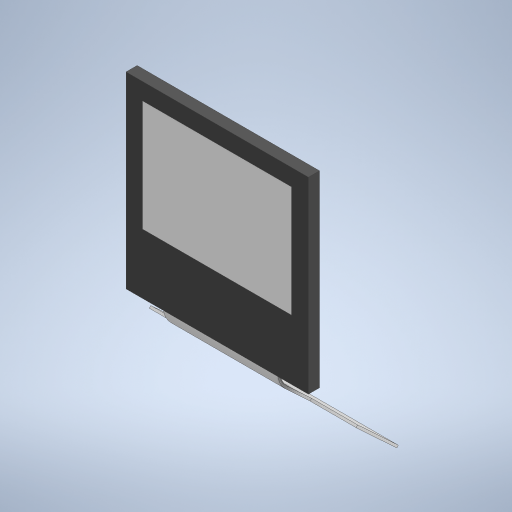
# Autodesk Inventor part: 0_42_oled
Saved by Autodesk Inventor 2023 (Build 270158000, 158)
## iProperties
Created: 2024-03-19
Part Number: 0_42_oled
Material: Generic
Document SubType Name: Modeling
Designer: noname
Density: 1 g/cm^3
Appearance: Default
Author: noname
Autodesk Inventor part; units mm, degrees
ref_plane "YZ Plane" through (0, 0, 0) normal (1, 0, 0) x (0, 1, 0)
ref_plane "XZ Plane" through (0, 0, 0) normal (0, 1, 0) x (-1, 0, 0)
ref_plane "XY Plane" through (0, 0, 0) normal (0, 0, 1) x (1, 0, 0)
sketch "Sketch2" plane through (0, 0, 0) normal (0, 0, 1) x (1, 0, 0)
  line L0 (-8.2, 0) -> (8.2, 0)
  line L1 (8.2, 0) -> (8.2, 16.9)
  line L2 (8.2, 16.9) -> (-8.2, 16.9)
  line L3 (-8.2, 16.9) -> (-8.2, 0)
  point P0 (0, 0)
  point P1 (0, 0)
  dimension "d0" = 16.4
  dimension "d1" = 16.9
  constraints: 8 end point, 2 parallel, 1 coincident, 1 horizontal, 1 midpoint, 1 perpendicular
  measures "d0" distance between parallel lines of L1 L3
  measures "d1" distance between parallel lines of L0 L2
extrude "Extrusion1" add sketch "Sketch2" along normal blind 1
ref_plane "Work Plane1" through (0, 0, 0.25) normal (0, 0, -1) x (-1, 0, 0)
sketch "Sketch5" plane through (0, 0, 0) normal (0, 0, -1) x (-1, 0, 0)
  line L0 (-6.7, 5.4) -> (6.7, 5.4)
  line L1 (6.7, 5.4) -> (6.7, 15.4)
  line L2 (6.7, 15.4) -> (-6.7, 15.4)
  line L3 (-6.7, 15.4) -> (-6.7, 5.4)
  line L4 (8.2, 16.9) -> (8.2, 0) projected
  line L5 (8.2, 0) -> (-8.2, 0) projected
  line L6 (-8.2, 16.9) -> (8.2, 16.9) projected
  point P0 (0, 0)
  point P1 (0, 5.4)
  point P2 (0, 0)
  dimension "d13" = 10
  dimension "d15" = 1.5
  dimension "d16" = 1.5
  constraints: 8 end point, 2 midpoint, 2 parallel, 1 horizontal, 1 perpendicular, 1 vertical alignment
  measures "d13" distance between parallel lines of L2 L0
  measures "d15" distance between parallel lines of L4 L1
  measures "d16" distance between parallel lines of L6 L2
ref_plane "Work Plane2" through (0, 0, 0) normal (1, 0, 0) x (0, 0, -1)
sketch "Sketch7" plane through (0, 0, 0) normal (1, 0, 0) x (0, 0, -1)
  arc A0 (-0.5, 0) -> (0.136, -1.4627) centre (1.5, 0) ccw
  line L0 (0, 0) -> (-1, 0) projected
  line L1 (0.136, -1.4627) -> (5.9868, -6.9187)
  line L2 (0, 16.9) -> (0, 0) projected
  line L3 (5.8504, -7.065) -> (-0.0004, -1.609)
  arc A1 (-0.7, 0) -> (-0.0004, -1.609) centre (1.5, 0) ccw
  line L4 (5.8504, -7.065) -> (5.9868, -6.9187)
  point P0 (5.9186, -6.9918)
  dimension "d19" = 2
  dimension "d22" = 43
  dimension "d23" = 0.5
  dimension "d24" = 0.2
  dimension "d33" = 8
  constraints: 6 end point, 4 point on circle, 2 centre point, 2 midpoint, 1 line through centre, 1 perpendicular, 1 point on line, 1 tangent, 1 other
  measures "d19" radius of A0
  measures "d22" angle of L0 L1
  measures "d23" distance from line of L2 A0.start
  measures "d24" distance between parallel lines of L1 L3
  measures "d33" distance of L1.start L1.end
extrude "Extrusion4" add sketch "Sketch7" along normal mid plane 10.3
sketch "Sketch8" plane through (0, 0, 0) normal (1, 0, 0) x (0, 0, -1)
  arc A0 (-0.5, 0) -> (0.136, -1.4627) centre (1.5, 0) ccw projected
  line L0 (-0.7, 0) -> (-0.5, 0) projected
  arc A1 (-0.7, 0) -> (-0.0004, -1.609) centre (1.5, 0) ccw construction
  line L1 (-0.0004, -1.609) -> (5.8504, -7.065) projected
  line L2 (5.8504, -7.065) -> (5.9868, -6.9187) projected
  line L3 (5.9868, -6.9187) -> (0.136, -1.4627) projected
  line L4 (2.1937, -3.655) -> (2.3301, -3.5087)
  point P0 (0, 0)
  dimension "d28" = 5
  constraints: 2 end point, 2 point on line, 1 perpendicular
  measures "d28" distance between parallel lines of L2 L4
extrude "Extrusion5" add sketch "Sketch8" along normal mid plane 18.6
sketch "Sketch9" plane through (0, 0, 1) normal (0, 0, 1) x (1, 0, 0)
  line L0 (6.7, 15.4) -> (6.7, 5.4) projected
  line L1 (6.7, 5.4) -> (-6.7, 5.4) projected
  line L2 (-6.7, 5.4) -> (-6.7, 15.4) projected
  line L3 (-6.7, 15.4) -> (6.7, 15.4) projected
  point P0 (0, 0)
extrude "Extrusion6" add sketch "Sketch9" along normal blind 0.01
equation "\"BendRadius\" = Thickness"
equation "\"BendReliefWidth\" = Thickness"
equation "\"BendReliefDepth\" = 0.5 * Thickness"
equation "\"CornerReliefSize\" = 4 * Thickness"
equation "\"MinimumRemnant\" = 2 * Thickness"
equation "\"TransitionRadius\" = BendRadius"
equation "\"JacobiRadiusSize\" = BendRadius"
equation "\"GapSize\" = Thickness"
equation "\"Thickness\" = 0.2"
body "Solid1"
